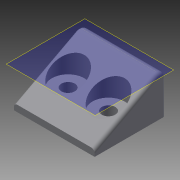
# Autodesk Inventor part: Anderson Holder
Saved by Autodesk Inventor 2015 (Build 190159000, 159)
## iProperties
Created: 2015-02-09
Part Number: Anderson Holder
Material: Generic
Document SubType Name: Modeling
Designer: whitaus15
Density: 1 g/cm^3
Appearance: Default
Author: whitaus15
Autodesk Inventor part; units mm, degrees
ref_plane "YZ Plane" through (0, 0, 0) normal (1, 0, 0) x (0, 1, 0)
ref_plane "XZ Plane" through (0, 0, 0) normal (0, 1, 0) x (-1, 0, 0)
ref_plane "XY Plane" through (0, 0, 0) normal (0, 0, 1) x (1, 0, 0)
sketch "Sketch1" plane through (0, 0, 0) normal (1, 0, 0) x (0, 1, 0)
  line L0 (0, 0) -> (15.3204, -29.0422)
  line L1 (12.5122, -33.6986) -> (0, -33.6986)
  line L2 (0, 0) -> (-3.0316, 0)
  line L3 (-3.0316, 0) -> (-3.0316, -33.6986)
  line L4 (-3.0316, -33.6986) -> (0, -33.6986)
  arc A0 (12.5122, -33.6986) -> (15.3204, -29.0422) centre (12.5122, -30.5236) ccw
  point P0 (17.7768, -33.6986)
  dimension "d0" = 38.1
  dimension "d1" = 3.175
  constraints: 10 end point, 2 horizontal, 2 perpendicular, 2 point on circle, 2 point on line, 2 tangent, 1 centre point
  measures "d0" distance of L0.start point (17.777, -33.699)
  measures "d1" radius of A0
extrude "Extrusion1" add sketch "Sketch1" along normal blind 38.1
fillet "Fillet1" radius 1.5875 8 edges at (38.1, 15.231, -32.1633) (38.1, 6.2561, -33.6986) (38.1, -1.5158, -33.6986) (38.1, 7.6602, -14.5211) (0, 15.231, -32.1633) (0, 6.2561, -33.6986) (0, -1.5158, -33.6986) (0, 7.6602, -14.5211)
sketch "Sketch2" plane through (0, -3.0316, 0) normal (0, -1, 0) x (1, 0, 0)
  line L0 (0, -32.1111) -> (0, 0) projected
  line L1 (0, -16.0556) -> (19.05, -16.0556)
  line L2 (19.05, -16.0556) -> (9.525, -16.0556)
  line L3 (19.05, -16.0556) -> (28.575, -16.0556)
  circle A0 centre (9.525, -16.0556) radius 3.175
  circle A1 centre (28.575, -16.0556) radius 3.175
  dimension "d5" = 19.05
  dimension "d6" = 9.525
  dimension "d7" = 6.35
  dimension "d8" = 6.35
  constraints: 6 end point, 2 centre point, 2 coincident, 2 midpoint, 1 horizontal, 1 point on line
  measures "d5" distance of L1.start L1.end
  measures "d6" distance of L1.end L3.end
  measures "d7" diameter of A0
  measures "d8" diameter of A1
extrude "Extrusion2" cut sketch "Sketch2" against normal blind 38.1
ref_plane "Work Plane1" through (0, 15.6872, -30.5236) normal (0, -1, 0) x (1, 0, 0)
sketch "Sketch3" plane through (0, 15.6872, -30.5236) normal (0, -1, 0) x (1, 0, 0)
  circle A0 centre (9.525, 14.4681) radius 3.175 projected
  circle A1 centre (28.575, 14.4681) radius 3.175 projected
  circle A2 centre (9.525, 14.4681) radius 7.62
  circle A3 centre (28.575, 14.4681) radius 7.62
  point P0 (0, 30.5236)
  dimension "d11" = 15.24
  dimension "d12" = 15.24
  constraints: 2 centre point, 2 coincident
  measures "d11" diameter of A2
  measures "d12" diameter of A3
extrude "Extrusion3" cut sketch "Sketch3" along normal blind 12.7
body "Solid1"
